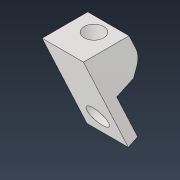
# Autodesk Inventor part: Ballsensor Platinenwinkel
Saved by Autodesk Inventor 2022.1 (Build 261234020, 234B)
## iProperties
Part Number: Ballsensor Platinenwinkel
Material: PC/ABS-Kunststoff
Document SubType Name: Modeling
Designer: rYan
Density: 0.357273 g/cm^3
Appearance: Glatt - Weiß
Mass: 0.0269362 g
Surface Area: 1.69373 cm^2
Volume: 0.075394 cm^3
Author: rYan
Autodesk Inventor part; units mm, degrees
ref_plane "YZ Plane" through (0, 0, 0) normal (1, 0, 0) x (0, 1, 0)
ref_plane "XZ Plane" through (0, 0, 0) normal (0, 1, 0) x (-1, 0, 0)
ref_plane "XY Plane" through (0, 0, 0) normal (0, 0, 1) x (1, 0, 0)
sketch "Skizze1" plane through (0, 0, 0) normal (1, 0, 0) x (0, 1, 0)
  line L0 (-1.5214, 0) -> (-5.9349, 0)
  line L1 (-5.9349, 0) -> (-1.5967, -9.3035)
  line L2 (0, -3.2627) -> (-1.5214, 0)
  line L3 (0, -3.2627) -> (-2.7189, -4.5306)
  line L4 (-2.7189, -4.5306) -> (-0.6904, -8.8808)
  line L5 (-0.6904, -8.8808) -> (-1.5967, -9.3035)
  line L6 (0, 1.8607) -> (0, -11.1642) projected
  point P0 (0, 0)
  dimension "d0" = 65
  dimension "d32" = 1
  dimension "d33" = 3
  dimension "d35" = 3.6
  dimension "d36" = 8.4
  constraints: 12 end point, 3 perpendicular, 2 point on line, 1 horizontal, 1 parallel
  measures "d0" angle of L1 L0
  measures "d32" distance of L4.end L1.end
  measures "d33" distance of L2.start L3.end
  measures "d35" distance of L2.start L0.start
  measures "d36" distance from line of L0.start L5
extrude "Extrusion1" add sketch "Skizze1" along normal mid plane 4
sketch "Skizze2" plane through (-2, -5.9349, 0) normal (0, 0, 1) x (1, 0, 0)
  line L0 (0, 0) -> (4, 0) projected
  line L1 (4, 4.4135) -> (4, 0) projected
  line L2 (4, 4.4135) -> (0, 4.4135) projected
  line L3 (0, 0) -> (0, 4.4135) projected
  line L4 (0, 4.3383) -> (0, 0) construction
  point P0 (2, 5.9349)
  point P1 (0, 4.7343)
  point P2 (2, 3.0135)
  dimension "d5" = 2
  dimension "d25" = 1.4
  measures "d5" distance from line of L3 point (2, 3.014)
  measures "d25" distance from line of L2 point (2, 3.014)
hole "Bohrung1" at (0, -2.9214, 0) direction (0, 0, -1) diameter 1.9 depth 3.4
sketch "Skizze3" plane through (-2, -1.8641, -8.7299) normal (0, -0.9063078, -0.4226183) x (1, 0, 0)
  line L0 (4, 9.6324) -> (4, -0.6329) projected
  line L1 (0, 9.6324) -> (4, 9.6324) projected
  line L2 (0, -0.6329) -> (0, 9.6324) projected
  line L3 (0, -0.6329) -> (4, -0.6329) projected
  point P0 (2, 1.6324)
  dimension "d26" = 2
  dimension "d29" = 8
  measures "d26" distance from line of point (2, 1.632) L0
  measures "d29" distance from line of L1 point (2, 1.632)
hole "Bohrung2" at (0, -2.554, -7.2505) direction (0, 0.9063078, 0.4226183) diameter 2.1 end through all
chamfer "Fase1" distance 1.2 angle 45 1 edges at (0, 0, -3.2627)
fillet "Rundung1" radius 2 1 edges at (0, -0.5071, -2.1751)
